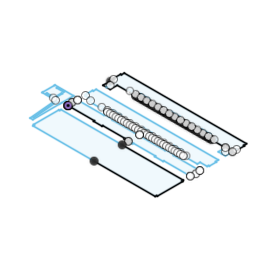
boitier_sysbee_decoupe (Autodesk Fusion 360 design; units mm, degrees)
Autodesk Fusion 360 part; units mm, degrees
sketch "Esquisse1" plane through (0, 0, 0) normal (0, 1, 0) x (1, 0, 0)
  line L0 (0, 0) -> (0, 7)
  line L1 (0, 7) -> (-3, 7)
  line L2 (-3, 7) -> (-3, 17)
  line L3 (0, 0) -> (93.75, 0)
  line L4 (93.75, 0) -> (93.75, -3)
  line L5 (93.75, -3) -> (123.75, -3)
  line L6 (123.75, -3) -> (123.75, 0)
  line L7 (123.75, 0) -> (202.5, 0)
  line L8 (202.5, 0) -> (202.5, -3)
  line L9 (202.5, -3) -> (217.5, -3)
  line L10 (202.5, 37) -> (217.5, 37)
  line L11 (-3, 27) -> (-3, 17)
  line L12 (202.5, 34) -> (202.5, 37)
  line L13 (123.75, 34) -> (202.5, 34)
  line L14 (0, 34) -> (0, 27)
  line L15 (0, 27) -> (-3, 27)
  line L16 (123.75, 37) -> (123.75, 34)
  line L17 (93.75, 37) -> (123.75, 37)
  line L18 (0, 34) -> (93.75, 34)
  line L19 (93.75, 34) -> (93.75, 37)
  line L20 (438, 7) -> (438, 17)
  line L21 (438, 27) -> (438, 17)
  line L22 (341.25, 37) -> (311.25, 37)
  line L23 (435, 34) -> (341.25, 34)
  line L24 (341.25, 0) -> (341.25, -3)
  line L25 (435, 27) -> (438, 27)
  line L26 (341.25, 34) -> (341.25, 37)
  line L27 (311.25, -3) -> (311.25, 0)
  line L28 (341.25, -3) -> (311.25, -3)
  line L29 (435, 34) -> (435, 27)
  line L30 (232.5, 34) -> (232.5, 37)
  line L31 (435, 0) -> (341.25, 0)
  line L32 (311.25, 0) -> (232.5, 0)
  line L33 (435, 7) -> (438, 7)
  line L34 (311.25, 37) -> (311.25, 34)
  line L35 (232.5, 0) -> (232.5, -3)
  line L36 (435, 0) -> (435, 7)
  line L37 (311.25, 34) -> (232.5, 34)
  line L38 (232.5, 37) -> (217.5, 37)
  line L39 (232.5, -3) -> (217.5, -3)
  point P0 (0, 34)
  point P1 (435, 34)
  point P2 (217.5, 37)
  point P3 (435, 0)
  dimension "d14" = 7
  dimension "plop" = 3
  dimension "d16" = 10
  dimension "d17" = 93.75
  dimension "d18" = 3
  dimension "d19" = 30
  dimension "d20" = 3
  dimension "d21" = 78.75
  dimension "d22" = 3
  dimension "d23" = 15
  constraint coincident L0.start L3.start
  constraint vertical L0
  constraint perpendicular L0 L1
  constraint perpendicular L1 L2
  constraint perpendicular L0 L3
  constraint perpendicular L3 L4
  constraint perpendicular L4 L5
  constraint perpendicular L5 L6
  constraint perpendicular L6 L7
  constraint perpendicular L7 L8
  constraint perpendicular L8 L9
  measures "d14" distance of L0.start L0.end
  measures "plop" distance of L0.end L1.end
  measures "d16" distance of L1.end L2.end
  measures "d17" distance of L0.start L3.end
  measures "d18" distance of L3.end L4.end
  measures "d19" distance of L4.end L5.end
  measures "d20" distance of L5.end L6.end
  measures "d21" distance of L6.end L7.end
  measures "d22" distance of L7.end L8.end
  measures "d23" distance of L8.end L9.end
sketch "Esquisse2" plane through (0, 0, 0) normal (0, 1, 0) x (1, 0, 0)
  line L0 (0, 60) -> (25, 60)
  line L1 (25, 60) -> (25, 50)
  line L2 (410, 50) -> (410, 60)
  line L3 (410, 60) -> (435, 60)
  line L4 (435, 60) -> (435, 65)
  line L5 (435, 65) -> (438, 65)
  line L6 (438, 65) -> (438, 90)
  line L7 (438, 90) -> (435, 90)
  line L8 (435, 90) -> (435, 100)
  line L9 (435, 100) -> (0, 100)
  line L10 (0, 100) -> (0, 90)
  line L11 (0, 90) -> (-3, 90)
  line L12 (-3, 90) -> (-3, 65)
  line L13 (-3, 65) -> (0, 65)
  line L14 (0, 65) -> (0, 60)
  line L15 (-3, 65) -> (0, 65)
  line L16 (0, 60) -> (0, 62) construction
  line L17 (93.75, 62) -> (93.75, 65)
  line L18 (93.75, 65) -> (123.75, 65)
  line L19 (123.75, 65) -> (123.75, 62)
  line L20 (123.75, 62) -> (93.75, 62)
  line L21 (25, 50) -> (25, 55) construction
  line L22 (60, 55) -> (60, 50)
  line L23 (70, 55) -> (70, 50)
  arc A0 (70, 55) -> (60, 55) centre (65, 55) ccw
  arc A1 (90, 55) -> (80, 55) centre (85, 55) ccw
  line L24 (90, 55) -> (90, 50)
  line L25 (80, 55) -> (80, 50)
  arc A2 (110, 55) -> (100, 55) centre (105, 55) ccw
  line L26 (110, 55) -> (110, 50)
  line L27 (100, 55) -> (100, 50)
  arc A3 (130, 55) -> (120, 55) centre (125, 55) ccw
  line L28 (130, 55) -> (130, 50)
  line L29 (120, 55) -> (120, 50)
  arc A4 (150, 55) -> (140, 55) centre (145, 55) ccw
  line L30 (150, 55) -> (150, 50)
  line L31 (140, 55) -> (140, 50)
  arc A5 (170, 55) -> (160, 55) centre (165, 55) ccw
  line L32 (170, 55) -> (170, 50)
  line L33 (160, 55) -> (160, 50)
  arc A6 (190, 55) -> (180, 55) centre (185, 55) ccw
  line L34 (190, 55) -> (190, 50)
  line L35 (180, 55) -> (180, 50)
  arc A7 (210, 55) -> (200, 55) centre (205, 55) ccw
  line L36 (210, 55) -> (210, 50)
  line L37 (200, 55) -> (200, 50)
  arc A8 (230, 55) -> (220, 55) centre (225, 55) ccw
  line L38 (230, 55) -> (230, 50)
  line L39 (220, 55) -> (220, 50)
  arc A9 (250, 55) -> (240, 55) centre (245, 55) ccw
  line L40 (250, 55) -> (250, 50)
  line L41 (240, 55) -> (240, 50)
  arc A10 (270, 55) -> (260, 55) centre (265, 55) ccw
  line L42 (270, 55) -> (270, 50)
  line L43 (260, 55) -> (260, 50)
  arc A11 (290, 55) -> (280, 55) centre (285, 55) ccw
  line L44 (290, 55) -> (290, 50)
  line L45 (280, 55) -> (280, 50)
  arc A12 (310, 55) -> (300, 55) centre (305, 55) ccw
  line L46 (310, 55) -> (310, 50)
  line L47 (300, 55) -> (300, 50)
  arc A13 (330, 55) -> (320, 55) centre (325, 55) ccw
  line L48 (330, 55) -> (330, 50)
  line L49 (320, 55) -> (320, 50)
  arc A14 (350, 55) -> (340, 55) centre (345, 55) ccw
  line L50 (350, 55) -> (350, 50)
  line L51 (340, 55) -> (340, 50)
  arc A15 (370, 55) -> (360, 55) centre (365, 55) ccw
  line L52 (370, 55) -> (370, 50)
  line L53 (360, 55) -> (360, 50)
  line L54 (202.5, 65) -> (232.5, 65)
  line L55 (202.5, 62) -> (202.5, 65)
  line L56 (232.5, 62) -> (202.5, 62)
  line L57 (232.5, 65) -> (232.5, 62)
  line L58 (311.25, 65) -> (341.25, 65)
  line L59 (311.25, 62) -> (311.25, 65)
  line L60 (341.25, 62) -> (311.25, 62)
  line L61 (341.25, 65) -> (341.25, 62)
  line L62 (25, 50) -> (60, 50)
  line L63 (70, 50) -> (80, 50)
  line L64 (90, 50) -> (100, 50)
  line L65 (110, 50) -> (120, 50)
  line L66 (130, 50) -> (140, 50)
  line L67 (150, 50) -> (160, 50)
  line L68 (170, 50) -> (180, 50)
  line L69 (190, 50) -> (200, 50)
  line L70 (210, 50) -> (220, 50)
  line L71 (230, 50) -> (240, 50)
  line L72 (250, 50) -> (260, 50)
  line L73 (270, 50) -> (280, 50)
  line L74 (290, 50) -> (300, 50)
  line L75 (310, 50) -> (320, 50)
  line L76 (330, 50) -> (340, 50)
  line L77 (350, 50) -> (360, 50)
  line L78 (370, 50) -> (410, 50)
  dimension "d28" = 25
  dimension "d29" = 10
  dimension "d30" = 385
  dimension "d31" = 25
  dimension "d32" = 5
  dimension "d33" = 3
  dimension "d34" = 25
  dimension "d36" = 10
  dimension "d37" = 435
  dimension "d38" = 10
  dimension "d39" = 3
  dimension "d40" = 25
  dimension "d43" = 2
  dimension "d44" = 93.75
  dimension "d45" = 3
  dimension "d46" = 30
  dimension "d56" = 5
  dimension "d57" = 40
  dimension "d76" = 20
  dimension "d77" = 0
  dimension "d79" = 5
  dimension "d80" = 10
  dimension "d83" = 108.75
  dimension "d84" = 0
  dimension "d87" = 20
  dimension "d88" = 0
  dimension "d89" = 10
  constraint perpendicular L0 L1
  constraint perpendicular L2 L3
  constraint perpendicular L3 L4
  constraint perpendicular L4 L5
  constraint perpendicular L5 L6
  constraint perpendicular L6 L7
  constraint perpendicular L7 L8
  constraint perpendicular L6 L9
  constraint perpendicular L7 L10
  constraint perpendicular L10 L11
  constraint perpendicular L7 L12
  constraint perpendicular L10 L13
  constraint perpendicular L0 L14
  constraint perpendicular L0 L16
  constraint perpendicular L17 L18
  constraint perpendicular L18 L19
  constraint perpendicular L22 L62
  constraint perpendicular L23 L63
  constraint horizontal L63
  constraint perpendicular L2 L78
  constraint horizontal L9
  constraint horizontal L17.start L19.end
  constraint vertical L4.end L7.end
  measures "d28" distance of L0.start L0.end
  measures "d29" distance of L0.end L1.end
  measures "d30" distance of L1.end L2.start
  measures "d31" distance of L2.end L3.end
  measures "d32" distance of L3.end L4.end
  measures "d33" distance of L4.end L5.end
  measures "d34" distance of L5.end L6.end
  measures "d36" distance of L7.end L8.end
  measures "d37" distance of L8.end L9.end
  measures "d38" distance of L9.end L10.end
  measures "d39" distance of L10.end L11.end
  measures "d40" distance of L11.end L12.end
  measures "d43" distance of L0.start L16.end
  measures "d44" distance of L16.end L17.start
  measures "d45" distance of L17.start L17.end
  measures "d46" distance of L17.end L18.end
  measures "d56" distance of L1.end L21.end
  measures "d57" distance of L21.end A0.centre
  measures "d79" distance of L23.start A0.centre
  measures "d80" distance of L22 L23
  measures "d89" distance of L2.start L2.end
sketch "face_laterale_boitier" plane through (0, 0, 0) normal (0, 1, 0) x (1, 0, 0)
  line L0 (-20, -3) -> (-20, 37)
  line L1 (-86.5, 37) -> (-86.5, -3)
  line L2 (-50, 7) -> (-47, 7)
  line L3 (-47, 7) -> (-47, 27)
  line L4 (-47, 27) -> (-50, 27)
  line L5 (-50, 27) -> (-50, 7)
  line L6 (-50, 34) -> (-75, 34)
  line L7 (-75, 34) -> (-75, 37)
  line L8 (-50, 0) -> (-75, 0)
  line L9 (-75, 0) -> (-75, -3)
  line L10 (-50, 34) -> (-50, 37)
  line L11 (-50, 0) -> (-50, -3)
  line L12 (-20, 37) -> (-20, 40)
  line L13 (-20, 40) -> (-86.5, 40)
  line L14 (-86.5, 40) -> (-86.5, 37)
  line L15 (-20, -3) -> (-20, -9.6961)
  line L16 (-86.5, -6) -> (-86.5, -3)
  line L17 (-75, 37) -> (-50, 37)
  line L18 (-75, -3) -> (-50, -3)
  line L19 (-20, -9.6961) -> (-19.417, -105.9984)
  line L20 (-23.4041, -97.5414) -> (-26.391, -97.8209)
  line L21 (-26.391, -97.8209) -> (-34.7776, -8.2125)
  line L22 (-34.7776, -8.2125) -> (-31.7907, -7.933)
  line L23 (-31.7907, -7.933) -> (-23.4041, -97.5414)
  line L24 (-29.1355, -106.0572) -> (-38.5, -6)
  line L25 (-19.417, -105.9984) -> (-29.1355, -106.0572)
  line L26 (-86.5, -6) -> (-38.5, -6)
  line L27 (-50, -3) -> (-50, 0)
  line L28 (-50, 0) -> (-75, 0)
  line L29 (-75, -3) -> (-50, -3)
  line L30 (-75, 0) -> (-75, -3)
  dimension "d169" = 40
  dimension "d170" = 66.5
  dimension "d175" = 40
  dimension "d176" = 20
  dimension "d184" = 25
  dimension "d185" = 3
  dimension "d186" = 3
  dimension "d243" = 3
  dimension "d245" = 3
  dimension "d246" = 90
  dimension "d255" = 3
  dimension "d271" = 103
  dimension "d272" = 3.5
  dimension "d275" = 95.347
  dimension "d279" = 48
  constraint vertical L5
  constraint vertical L3
  constraint parallel L7 L10
  constraint perpendicular L6 L10
  constraint horizontal L10.end L7.end
  constraint perpendicular L12 L13
  constraint vertical L16
  constraint parallel L21 L23
  constraint parallel L20 L22
  constraint perpendicular L1 L13
  constraint perpendicular L13 L14
  constraint parallel L21 L24
  constraint perpendicular L19 L25
  constraint coincident L24 L26.end
  constraint perpendicular L16 L26
  constraint parallel L13 L26
  measures "d169" distance of L0.start L0.end
  measures "d170" distance of L0.end L1.start
  measures "d175" distance of L11.end L10.end
  measures "d176" distance of L2.end L3.end
  measures "d184" distance of L6.start L6.end
  measures "d185" distance of L10.end L6.start
  measures "d186" distance of L0.end L12.end
  measures "d243" distance of L1.end L16.start
  measures "d245" distance of L20.start L20.end
  measures "d246" distance of L20.start L22.end
  measures "d255" distance of L1.start L13.end
  measures "d271" distance of L0.start L19.end
  measures "d272" distance of L21 L24
  measures "d275" angle of L24 L26
  measures "d279" distance of L16.start L24.end
extrude "Extrude1" add sketch "face_laterale_boitier" along normal blind 3 makes body 1
extrude "Extrude2" add sketch "Esquisse2" along normal blind 3 separate body makes body 2
extrude "Extrude3" add sketch "Esquisse1" along normal blind 3 separate body makes body 3
copy_body "Body->Comp1" bodies 1 removing the originals makes body 4 in component "face_gauche"
copy_body "Body->Comp1'" bodies 4 removing the originals makes body 5 in component "face_gauche (1)"
copy_body "Body->Comp2" bodies 2 removing the originals makes body 6 in component "face_arriere"
copy_body "Body->Comp3" bodies 3 removing the originals makes body 7 in component "support_carte"
extrude "Extrude1'" add sketch "Esquisse2" along normal blind 3 separate body makes body 8 in component "face_avant"
extrude "Extrude1''" add sketch "face_laterale_boitier" along normal blind 3 separate body makes body 9 in component "face_droite"
sketch "planche_envol" plane through (0, 0, 0) normal (0, 1, 0) x (1, 0, 0)
  line L0 (-3, -30) -> (0, -30)
  line L1 (0, -30) -> (0, -25)
  line L2 (0, -25) -> (217.5, -25)
  line L3 (-3, -30) -> (-3, -120)
  line L4 (-3, -120) -> (0, -120)
  line L5 (0, -120) -> (0, -125)
  line L6 (0, -125) -> (217.5, -125)
  line L7 (435, -25) -> (217.5, -25)
  line L8 (435, -30) -> (435, -25)
  line L9 (438, -30) -> (435, -30)
  line L10 (438, -30) -> (438, -120)
  line L11 (438, -120) -> (435, -120)
  line L12 (435, -120) -> (435, -125)
  line L13 (435, -125) -> (217.5, -125)
  dimension "d257" = 3
  dimension "d258" = 5
  dimension "d259" = 217.5
  dimension "d260" = 90
  dimension "d261" = 3
  dimension "d262" = 5
  dimension "d264" = 25
  constraint horizontal L0
  constraint perpendicular L0 L1
  constraint perpendicular L1 L2
  constraint perpendicular L0 L3
  constraint perpendicular L3 L4
  constraint perpendicular L0 L5
  constraint perpendicular L5 L6
  constraint equal L2 L6
  measures "d257" distance of L0.start L0.end
  measures "d258" distance of L0.end L1.end
  measures "d259" distance of L1.end L2.end
  measures "d260" distance of L0.start L3.end
  measures "d261" distance of L3.end L4.end
  measures "d262" distance of L4.end L5.end
  measures "d264" distance of origin L1.end
extrude "Extrude1'''" add sketch "planche_envol" along normal blind 3 separate body makes body 10 in component "planche_envol"
sketch "face_avant_boitier" plane through (0, 0, 0) normal (0, 1, 0) x (1, 0, 0)
  line L0 (340, 155) -> (340, 150)
  line L1 (123.75, 165) -> (123.75, 162)
  line L2 (320, 155) -> (320, 150)
  arc A0 (110, 155) -> (100, 155) centre (105, 155) ccw
  line L3 (90, 150) -> (100, 150)
  line L4 (90, 155) -> (90, 150)
  line L5 (202.5, 165) -> (232.5, 165)
  line L6 (190, 150) -> (200, 150)
  line L7 (300, 155) -> (300, 150)
  line L8 (130, 150) -> (140, 150)
  line L9 (310, 150) -> (320, 150)
  line L10 (290, 155) -> (290, 150)
  line L11 (60, 155) -> (60, 150)
  line L12 (190, 155) -> (190, 150)
  line L13 (160, 155) -> (160, 150)
  line L14 (80, 155) -> (80, 150)
  line L15 (25, 125) -> (25, 150)
  line L16 (120, 155) -> (120, 150)
  line L17 (232.5, 162) -> (202.5, 162)
  line L18 (330, 150) -> (340, 150)
  line L19 (341.25, 165) -> (341.25, 162)
  arc A1 (70, 155) -> (60, 155) centre (65, 155) ccw
  arc A2 (310, 155) -> (300, 155) centre (305, 155) ccw
  arc A3 (210, 155) -> (200, 155) centre (205, 155) ccw
  line L20 (150, 155) -> (150, 150)
  line L21 (330, 155) -> (330, 150)
  line L22 (370, 150) -> (410, 150)
  line L23 (0, 200) -> (0, 190)
  line L24 (0, 190) -> (-3, 190)
  line L25 (350, 155) -> (350, 150)
  line L26 (-3, 190) -> (-3, 165)
  line L27 (435, 165) -> (438, 165)
  line L28 (0, 125) -> (0, 162) construction
  line L29 (-3, 165) -> (0, 165)
  line L30 (0, 165) -> (0, 125)
  line L31 (438, 165) -> (438, 190)
  line L32 (93.75, 165) -> (123.75, 165)
  line L33 (435, 190) -> (435, 200)
  line L34 (438, 190) -> (435, 190)
  line L35 (310, 155) -> (310, 150)
  line L36 (0, 150) -> (0, 125) construction
  line L37 (311.25, 165) -> (341.25, 165)
  line L38 (350, 150) -> (360, 150)
  line L39 (-3, 165) -> (0, 165)
  arc A4 (230, 155) -> (220, 155) centre (225, 155) ccw
  line L40 (220, 155) -> (220, 150)
  line L41 (250, 150) -> (260, 150)
  line L42 (260, 155) -> (260, 150)
  line L43 (270, 150) -> (280, 150)
  arc A5 (290, 155) -> (280, 155) centre (285, 155) ccw
  line L44 (270, 155) -> (270, 150)
  line L45 (210, 150) -> (220, 150)
  line L46 (280, 155) -> (280, 150)
  line L47 (240, 155) -> (240, 150)
  line L48 (435, 200) -> (0, 200)
  line L49 (250, 155) -> (250, 150)
  line L50 (150, 150) -> (160, 150)
  arc A6 (150, 155) -> (140, 155) centre (145, 155) ccw
  line L51 (232.5, 165) -> (232.5, 162)
  line L52 (230, 150) -> (240, 150)
  arc A7 (270, 155) -> (260, 155) centre (265, 155) ccw
  line L53 (70, 150) -> (80, 150)
  line L54 (123.75, 162) -> (93.75, 162)
  arc A8 (170, 155) -> (160, 155) centre (165, 155) ccw
  line L55 (210, 155) -> (210, 150)
  arc A9 (250, 155) -> (240, 155) centre (245, 155) ccw
  line L56 (230, 155) -> (230, 150)
  arc A10 (130, 155) -> (120, 155) centre (125, 155) ccw
  arc A11 (90, 155) -> (80, 155) centre (85, 155) ccw
  line L57 (25, 150) -> (60, 150)
  line L58 (100, 155) -> (100, 150)
  line L59 (311.25, 162) -> (311.25, 165)
  line L60 (130, 155) -> (130, 150)
  line L61 (202.5, 162) -> (202.5, 165)
  line L62 (93.75, 162) -> (93.75, 165)
  line L63 (290, 150) -> (300, 150)
  line L64 (170, 155) -> (170, 150)
  line L65 (140, 155) -> (140, 150)
  line L66 (110, 150) -> (120, 150)
  line L67 (70, 155) -> (70, 150)
  arc A12 (190, 155) -> (180, 155) centre (185, 155) ccw
  line L68 (110, 155) -> (110, 150)
  line L69 (170, 150) -> (180, 150)
  arc A13 (330, 155) -> (320, 155) centre (325, 155) ccw
  line L70 (180, 155) -> (180, 150)
  line L71 (200, 155) -> (200, 150)
  line L72 (370, 155) -> (370, 150)
  line L73 (435, 150) -> (435, 165)
  line L74 (360, 155) -> (360, 150)
  arc A14 (350, 155) -> (340, 155) centre (345, 155) ccw
  arc A15 (370, 155) -> (360, 155) centre (365, 155) ccw
  line L75 (341.25, 162) -> (311.25, 162)
  line L76 (14, 137.5) -> (14, 125)
  line L77 (11, 137.5) -> (11, 125)
  arc A16 (14, 137.5) -> (11, 137.5) centre (12.5, 137.5) ccw
  line L78 (0, 125) -> (11, 125)
  line L79 (14, 125) -> (25, 125)
  line L80 (435, 165) -> (435, 125)
  line L81 (435, 125) -> (424, 125)
  line L82 (424, 137.5) -> (424, 125)
  line L83 (421, 137.5) -> (421, 125)
  arc A17 (424, 137.5) -> (421, 137.5) centre (422.5, 137.5) ccw
  line L84 (421, 125) -> (410, 125)
  line L85 (410, 125) -> (410, 150)
  point P0 (435, 150)
  dimension "d302" = 20
  dimension "d303" = 0
  dimension "d306" = 108.75
  dimension "d307" = 0
  dimension "d310" = 20
  dimension "d311" = 0
  dimension "d314" = 25
  dimension "d316" = 385
  dimension "d318" = 15
  dimension "d319" = 3
  dimension "d320" = 25
  dimension "d321" = 10
  dimension "d322" = 435
  dimension "d324" = 3
  dimension "d325" = 25
  dimension "d327" = 93.75
  dimension "d328" = 3
  dimension "d329" = 30
  dimension "d332" = 5
  dimension "d333" = 10
  dimension "d335" = 60
  dimension "d338" = 50
  dimension "d339" = 25
  dimension "d341" = 10
  dimension "d344" = 3
  dimension "d346" = 150
  constraint perpendicular L15 L78
  constraint perpendicular L27 L73
  constraint perpendicular L27 L31
  constraint perpendicular L31 L34
  constraint perpendicular L33 L34
  constraint perpendicular L31 L48
  constraint perpendicular L23 L34
  constraint perpendicular L23 L24
  constraint perpendicular L26 L34
  constraint perpendicular L23 L29
  constraint perpendicular L30 L78
  constraint perpendicular L28 L78
  constraint perpendicular L32 L62
  constraint perpendicular L1 L32
  constraint perpendicular L11 L57
  constraint perpendicular L53 L67
  constraint horizontal L53
  constraint horizontal L48
  constraint horizontal L1.end L54.end
  constraint vertical L33.start L27.start
  constraint vertical L36
  constraint horizontal L78
  constraint coincident L76.end L78
  constraint tangent L76 A16
  constraint perpendicular L76 L78
  constraint tangent L77 A16
  constraint perpendicular L77 L78
  constraint collinear L78 L79
  constraint horizontal L36.start L15.end
  constraint horizontal L22
  constraint vertical L33.end L80.end
  measures "d314" distance of L28.start L15.start
  measures "d316" distance of L15.end L22.end
  measures "d318" distance of P0 L27.start
  measures "d319" distance of L27.end L27.start
  measures "d320" distance of L27.end L31.end
  measures "d321" distance of L33.end L33.start
  measures "d322" distance of L23.start L33.end
  measures "d324" distance of L24.end L23.end
  measures "d325" distance of L24.end L26.end
  measures "d327" distance of L28.end L54.end
  measures "d328" distance of L32.start L54.end
  measures "d329" distance of L32.start L1.start
  measures "d332" distance of A1.start A1.centre
  measures "d333" distance of L11 L67
  measures "d335" distance of L11 L36
  measures "d338" distance of L23.start L36.start
  measures "d339" distance of L15.end L15.start
  measures "d341" distance of L23.start L23.end
  measures "d344" diameter of A16
  measures "d346" distance of origin L36.start
component "face_avant" placed x (1, 0, 0) y (0, 0, 1) z (0, -1, 0) at (0, -62, 0)
component "face_droite" placed x (0, -1, 0) y (1, 0, 0) z (0, 0, 1) at (435, -47, 0)
component "planche_envol" placed x (1, 0, 0) y (0, 0.995649, 0.093185) z (0, -0.093185, 0.995649) at (0, -12.4138, -21.9365)
component "face_gauche" placed x (1, 0, 0) y (0, 1, 0) z (0, 0, 1) at (0, 0, 0)
component "face_arriere" placed x (1, 0, 0) y (0, 0, 1) z (0, -1, 0) at (0, -62, -37)
component "support_carte" placed x (1, 0, 0) y (0, 1, 0) z (0, 0, 1) at (0, 0, 0)
component "face_gauche (1)" placed x (0, -1, 0) y (1, 0, 0) z (0, 0, 1) at (-3, -47, 0) in component "face_gauche"
equation "plop = epaisseur"
equation "d18 = epaisseur"
equation "d20 = epaisseur"
equation "d22 = plop"
equation "d30 = 435 mm - 50 mm"
equation "d33 = epaisseur"
equation "d39 = epaisseur"
equation "d45 = epaisseur"
equation "epaisseur = 3 mm" comment "épaisseur du bois"
equation "d169 = 34 mm + 2 * epaisseur"
equation "d175 = 34 mm + 2 * epaisseur"
equation "d185 = epaisseur"
equation "d188 = epaisseur"
equation "d190 = epaisseur"
equation "d192 = epaisseur"
equation "d229 = epaisseur"
equation "d231 = epaisseur"
equation "d245 = epaisseur"
equation "d257 = epaisseur"
equation "d259 = ( 435 / 2 ) * 1 mm"
equation "d261 = epaisseur"
equation "d265 = epaisseur"
equation "d316 = 435 mm - 50 mm"
equation "d319 = epaisseur"
equation "d324 = epaisseur"
equation "d328 = epaisseur"
named bodies: "face_gauche", "face_arriere", "support_carte"
